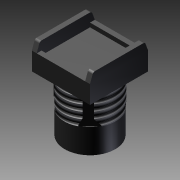
# Autodesk Inventor part: YB16SKW01-BBni_body
Saved by Autodesk Inventor 2015 SP1 (Build 190203100, 203)
## iProperties
Category: PARTsolutions
Company: NKKSWITCHES
Created: 2013-12-31
Part Number: YB16SKW01-BBni_body
Catalog Web Link: www.cadenas.de
Description: Panel Mount Non-Illuminated Pushbuttons_ni_body-
Vendor: NKKSWITCHES
Document SubType Name: Modeling
Designer: PARTuser1
Manufacturer: NKKSWITCHES
Density: 1 g/cm^3
Material: Generic
Appearance: RGB(0.00000000000000,0.00000000000000,0.00000000000000)
PSOL_IDENT_0: {$CADENAS_DATA\23d-libs\nkkswitches\pushbuttons\yb\parts\yb_ni_body.prj},254 {VTYP=3D},{NB=YB16SKW01
PSOL_IDENT_1: -BBni_body},{LINA=YB16SKW01-BBni_body},{NN=Panel Mount Non-Illuminated Pushbuttons_ni_body},{DATE=29
PSOL_IDENT_2: .03.2013 10:04:04},{GEOMDATE=29.03.2013 11:03:00},{VERSION=},{LINEID=10},{LINESUBID=-1},{WBVAR=PLS,C
PSOL_IDENT_3: RCTS,PS,SHPS,CMR,TRMNLS,CCLR}  {NB=YB16SKW01-BBni_body},{LINA=YB16SKW01-BBni_body},{KT=DUMMY},{PN=YB
PSOL_IDENT_4: 16SKW01-BB},{SRS=YB},{PLS=1},{CRCTS=6},{PS=},{SHPS=S},{SHPSALG= 'S', 'S - Square (Bushing Mounting)'
PSOL_IDENT_5: , 'C'  , 'C - Round (Bushing Mounting)', 'R', 'R - Rectangular (Bushing Mounting)'  , 'K', 'K - Squa
PSOL_IDENT_6: re (Snap-in Mounting)', 'M', 'M - Round (Snap-in Mounting)'  , 'N', 'N - Rectangular (Snap-in Mounti
PSOL_IDENT_7: ng)' },{HSNG=K - Black only},{CMR=W},{TRMNLS=01},{A=0.709},{A1=0.591},{A11=0.827},{B=0.709},{B1=0.59
PSOL_IDENT_8: 1},{L=0.669},{L1=0.327},{L2=0.957},{L3=0.429},{L4=0.370},{L5=0.118},{L6=0.209},{L7=0.157},{DIA1=0.59
PSOL_IDENT_9: 1},{DIA=0.709},{COL=0.75,0.75,0.75,0.00},{OCHR=Download pdf},{NDM=16.000},{CCLR=BB}
CNS_NN: Panel Mount Non-Illuminated Pushbuttons_ni_body
CNS_NB: YB16SKW01-BBni_body
CNS_NBSYN: $PN.ni_body
CNS_LINA: YB16SKW01-BBni_body
CNS_PN: YB16SKW01-BB
CNS_SRS: YB
CNS_PLS: 1 - SPDT
CNS_CRCTS: 6 - ON/ON
CNS_PS: Without Panel Seal
CNS_SHPS: S - Square (Bushing Mounting)
CNS_SHPSALG: 'S', 'S - Square (Bushing Mounting)', 'C'  , 'C - Round (Bushing Mounting)', 'R', 'R - Rectangular (Bushing Mounting)'  , 'K', 'K - Square (Snap-in Mounting)', 'M', 'M - Round (Snap-in Mounting)'  , 'N', 'N - Rectangular (Snap-in Mounting)'
CNS_HSNG: K - Black only
CNS_CMR: W - Silver; Rated 3A @ 125V AC
CNS_TRMNLS: 01 - Solder Lug/.110" (2.8mm) Quick Connect
CNS_A: 0.709
CNS_A1: 0.591
CNS_A11: 0.827
CNS_B: 0.709
CNS_B1: 0.591
CNS_L: 0.669
CNS_L1: 0.327
CNS_L2: 0.957
CNS_L3: 0.429
CNS_L4: 0.370
CNS_L5: 0.118
CNS_L6: 0.209
CNS_L7: 0.157
CNS_DIA1: 0.591
CNS_DIA: 0.709
CNS_COL: 0.75,0.75,0.75,0.00
CNS_OCHR: Download pdf
CNS_NDM: 16.000
CNS_CCLR: BB - White/White
SUPPLIER: NKKSWITCHES
ARTICLENO: YB16SKW01-BBni_body
BOMINFO: YB16SKW01-BBni_body
CREATOR: CADENAS GmbH
Title: YB16SKW01-BBni_body
Author: Cadenas PARTsolutions
Autodesk Inventor part; units mm, degrees
sketch "Sketch_1" plane through (0, 0, 0) normal (0, 0, 1) x (1, 0, 0)
  line L0 (0, 0) -> (0, -9.398)
  line L1 (0, -9.398) -> (-8, -9.398)
  line L2 (-8, -9.398) -> (-8, -0.8382)
  line L3 (-8, -0.8382) -> (-8.0808, -0.8382)
  line L4 (-8.0808, -0.8382) -> (-8.0808, 0)
  line L5 (-8.0808, 0) -> (0, 0)
  line L6 (0, 0) -> (0, -9.398)
  constraints: 14 end point
revolve "Revolution1" add sketch "Sketch_1" angle 360 about axis through (0, 0, 0) along (0, 1, 0)
thread "Thread1" size "M16x2" class "6g" standard "ISO Metric profile" full length
sketch "Sketch_15" plane through (0, 0, 0) normal (0, 0, 1) x (1, 0, 0)
  line L0 (0, -9.398) -> (0, -16.9926)
  line L1 (0, -16.9926) -> (-7.8049, -16.9926)
  line L2 (-7.8049, -16.9926) -> (-7.8049, -9.398)
  line L3 (-7.8049, -9.398) -> (0, -9.398)
  line L4 (0, -9.398) -> (0, -16.9926)
  constraints: 10 end point
revolve "Revolution2" add sketch "Sketch_15" angle 360 about axis through (0, -9.398, 0) along (0, 1, 0)
sketch "Sketch_7" plane through (-5.714, 0, 5.714) normal (0.7071, 0, -0.7071) x (-0.7071, 0, -0.7071)
  line L0 (-2.7242, -9.398) -> (2.7242, -9.398)
  line L1 (2.7242, -9.398) -> (0.9081, -7.2337)
  line L2 (0.9081, -7.2337) -> (0.9081, 0)
  line L3 (0.9081, 0) -> (-1.6345, 0)
  line L4 (-1.6345, 0) -> (-1.6345, -7.0612)
  line L5 (-1.6345, -7.0612) -> (-2.7242, -9.398)
  constraints: 12 end point
extrude "Extrusion1" cut sketch "Sketch_7" along normal blind 0.508
sketch "Sketch_9" plane through (5.714, 0, 5.714) normal (0.7071, 0, 0.7071) x (0.7071, 0, -0.7071)
  line L0 (-2.7242, -9.398) -> (2.7242, -9.398)
  line L1 (2.7242, -9.398) -> (0.9081, -7.2337)
  line L2 (0.9081, -7.2337) -> (0.9081, 0)
  line L3 (0.9081, 0) -> (-1.6345, 0)
  line L4 (-1.6345, 0) -> (-1.6345, -7.0612)
  line L5 (-1.6345, -7.0612) -> (-2.7242, -9.398)
  constraints: 12 end point
extrude "Extrusion2" cut sketch "Sketch_9" against normal blind 0.508
sketch "Sketch_8" plane through (5.714, 0, -5.714) normal (0.7071, 0, -0.7071) x (-0.7071, 0, -0.7071)
  line L0 (-2.7242, -9.398) -> (2.7242, -9.398)
  line L1 (2.7242, -9.398) -> (1.6345, -7.0612)
  line L2 (1.6345, -7.0612) -> (1.6345, 0)
  line L3 (1.6345, 0) -> (-0.9081, 0)
  line L4 (-0.9081, 0) -> (-0.9081, -7.2337)
  line L5 (-0.9081, -7.2337) -> (-2.7242, -9.398)
  constraints: 12 end point
extrude "Extrusion3" cut sketch "Sketch_8" against normal blind 0.508
sketch "Sketch_10" plane through (-5.714, 0, -5.714) normal (0.7071, 0, 0.7071) x (0.7071, 0, -0.7071)
  line L0 (-2.7242, -9.398) -> (2.7242, -9.398)
  line L1 (2.7242, -9.398) -> (1.6345, -7.0612)
  line L2 (1.6345, -7.0612) -> (1.6345, 0)
  line L3 (1.6345, 0) -> (-0.9081, 0)
  line L4 (-0.9081, 0) -> (-0.9081, -7.2337)
  line L5 (-0.9081, -7.2337) -> (-2.7242, -9.398)
  constraints: 12 end point
extrude "Extrusion4" cut sketch "Sketch_10" along normal blind 0.508
sketch "Sketch_14" plane through (-8.2051, 0, 0) normal (1, 0, 0) x (0, 0, -1)
  line L0 (-1.4346, -7.2187) -> (-0.8534, -7.9113)
  line L1 (-0.8534, -7.9113) -> (-0.8534, -9.398)
  line L2 (-0.8534, -9.398) -> (0.8534, -9.398)
  line L3 (0.8534, -9.398) -> (0.8534, -7.9113)
  line L4 (0.8534, -7.9113) -> (1.4346, -7.2187)
  line L5 (1.4346, -7.2187) -> (1.4346, 0)
  line L6 (1.4346, 0) -> (-1.4346, 0)
  line L7 (-1.4346, 0) -> (-1.4346, -7.2187)
  constraints: 16 end point
extrude "Extrusion5" cut sketch "Sketch_14" along normal blind 0.508
sketch "Sketch_20" plane through (0, 0, 0) normal (1, 0, 0) x (0, 1, 0)
  line L0 (0, 9.0043) -> (0, -9.0043)
  line L1 (0, -9.0043) -> (5.588, -9.0043)
  line L2 (5.588, -9.0043) -> (7.8044, -8.1976)
  arc A0 (7.8044, -8.1976) -> (8.3058, -7.4815) centre (7.5438, -7.4815) ccw
  line L3 (8.3058, -7.4815) -> (8.3058, 7.4815)
  arc A1 (8.3058, 7.4815) -> (7.8044, 8.1976) centre (7.5438, 7.4815) ccw
  line L4 (7.8044, 8.1976) -> (5.588, 9.0043)
  line L5 (5.588, 9.0043) -> (0, 9.0043)
  constraints: 12 end point, 4 point on circle, 2 centre point
extrude "Extrusion6" add sketch "Sketch_20" along normal mid plane 18.0086
sketch "Sketch_19" plane through (0, 0, 0) normal (0, 0, 1) x (1, 0, 0)
  line L0 (-7.5057, 5.588) -> (7.5057, 5.588)
  line L1 (7.5057, 5.588) -> (7.5057, 9.5758)
  line L2 (7.5057, 9.5758) -> (-7.5057, 9.5758)
  line L3 (-7.5057, 9.5758) -> (-7.5057, 5.588)
  constraints: 8 end point
extrude "Extrusion7" cut sketch "Sketch_19" along normal mid plane 30.0228
sketch "Sketch_18" plane through (0, 4.318, 0) normal (0, 1, 0) x (1, 0, 0)
  line L0 (-7.5057, 7.5057) -> (-7.5057, -7.5057)
  line L1 (-7.5057, -7.5057) -> (7.5057, -7.5057)
  line L2 (7.5057, -7.5057) -> (7.5057, 7.5057)
  line L3 (7.5057, 7.5057) -> (-7.5057, 7.5057)
  constraints: 8 end point
extrude "Extrusion8" cut sketch "Sketch_18" along normal blind 8.3058
sketch "Sketch_2" plane through (0, -16.9926, 0) normal (0, 1, 0) x (1, 0, 0)
  line L0 (-0.7, -6.096) -> (0.7, -6.096)
  line L1 (0.7, -6.096) -> (0.7, -4.896)
  line L2 (0.7, -4.896) -> (-0.7, -4.896)
  line L3 (-0.7, -4.896) -> (-0.7, -6.096)
  constraints: 8 end point
extrude "Extrusion9" add sketch "Sketch_2" along normal mid plane 2.6
ref_plane "body_to_cap_XY" through (0, 4.318, 0) normal (0, 1, 0) x (1, 0, 0)
ref_plane "body_to_cap_YZ" through (0, 4.318, 0) normal (1, 0, 0) x (0, 0, -1)
ref_plane "body_to_cap_ZX" through (0, 4.318, 0) normal (0, 0, -1) x (0, 1, 0)
ref_plane "body_to_metal_XY" through (0, -8.7173, 0) normal (0, 1, 0) x (1, 0, 0)
ref_plane "body_to_metal_YZ" through (0, -8.7173, 0) normal (1, 0, 0) x (0, 0, -1)
ref_plane "body_to_metal_ZX" through (0, -8.7173, 0) normal (0, 0, -1) x (0, 1, 0)
ref_plane "body_to_nut_XY" through (0, 0, 0) normal (0, 1, 0) x (1, 0, 0)
ref_plane "body_to_nut_YZ" through (0, 0, 0) normal (1, 0, 0) x (0, 0, -1)
ref_plane "body_to_nut_ZX" through (0, 0, 0) normal (0, 0, -1) x (0, 1, 0)
body "Solid1"
